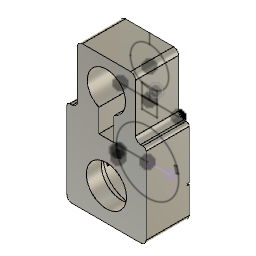
MotorEnclosure v3 (Autodesk Fusion 360 design; units mm, degrees)
Autodesk Fusion 360 part; units mm, degrees
sketch "Sketch1" plane through (0, 0, 0) normal (0, 0, 1) x (1, 0, 0)
  line L0 (-29, 0) -> (29, 0)
  line L1 (29, 0) -> (29, -17)
  line L2 (29, -17) -> (-29, -17)
  line L3 (-29, -17) -> (-29, 0)
  line L4 (-31, 2) -> (31, 2)
  line L5 (31, 2) -> (31, 0)
  line L6 (31, 0) -> (-31, 0)
  line L7 (-31, 0) -> (-31, 2)
  line L8 (-27.55, -17) -> (27.55, -17)
  line L9 (27.55, -17) -> (27.55, -26)
  line L10 (27.55, -26) -> (-27.55, -26)
  line L11 (-27.55, -26) -> (-27.55, -17)
  line L12 (-20, -26) -> (20, -26)
  line L13 (20, -26) -> (20, -41)
  line L14 (20, -41) -> (-20, -41)
  line L15 (-20, -41) -> (-20, -26)
  line L16 (-42.5, 22) -> (42.5, 22)
  line L17 (42.5, 22) -> (42.5, 2)
  line L18 (42.5, 2) -> (-42.5, 2)
  line L19 (-42.5, 2) -> (-42.5, 22)
  line L20 (-42.5, -41) -> (-20, -41)
  line L21 (42.5, 2) -> (42.5, 22)
  line L22 (-39.5, 2) -> (-39.5, -41)
  line L23 (20, -41) -> (39.5, -41)
  line L24 (39.5, -41) -> (39.5, 2)
  line L25 (0, 2) -> (0, 22)
  line L26 (0, 2) -> (0, -41)
  dimension "d1" = 17
  dimension "d2" = 58
  dimension "d3" = 2
  dimension "d4" = 62
  dimension "d5" = 55.1
  dimension "d6" = 9
  dimension "d7" = 15
  dimension "d8" = 40
  dimension "d9" = 85
  dimension "d10" = 20
  dimension "d23" = 3
  dimension "d24" = 3
  constraint horizontal L0
  constraint vertical L1
  constraint horizontal L2
  constraint vertical L3
  constraint horizontal L4
  constraint vertical L5
  constraint horizontal L6
  constraint vertical L7
  constraint midpoint origin L0
  constraint midpoint origin L6
  constraint horizontal L8
  constraint vertical L9
  constraint horizontal L10
  constraint vertical L11
  constraint coincident L2 L8.start
  constraint horizontal L12
  constraint vertical L13
  constraint horizontal L14
  constraint vertical L15
  constraint coincident L10 L12.start
  constraint horizontal L16
  constraint vertical L17
  constraint horizontal L18
  constraint vertical L19
  constraint collinear L4 L18
  constraint perpendicular L15 L20
  constraint vertical L21
  constraint coincident L18 L22.start
  constraint coincident L20 L22.end
  constraint perpendicular L20 L22
  constraint perpendicular L13 L23
  constraint coincident L18 L24.end
  constraint perpendicular L18 L24
  constraint midpoint L4 L25.start
  constraint midpoint L16 L25.end
  constraint perpendicular L4 L25
  constraint symmetric L13 L15 L25
  constraint symmetric L9 L11 L25
  constraint midpoint L14 L26.end
  measures "d1" distance of L0.start L2.end
  measures "d2" distance of L0.start L0.end
  measures "d3" distance of L4.start L6.end
  measures "d4" distance of L4.start L4.end
  measures "d5" distance of L9.end L10.end
  measures "d6" distance of L8.start L10.end
  measures "d7" distance of L12.start L14.end
  measures "d8" distance of L13.end L14.end
  measures "d9" distance of L17.end L18.end
  measures "d10" distance of L16.start L18.end
  measures "d23" distance of L19 L22
  measures "d24" distance of L21 L24
extrude "Extrude3" add sketch "Sketch1" along normal mid plane 65 contours L0 L4 L6 L7 L18 L26 | L0 L2 L3 L6 L8 L26 | L2 L3 L6 L7 L10 L11 L15 L18 L20 L22 | L0 L4 L5 L6 L18 L26 | L0 L1 L2 L6 L8 L26 | L1 L2 L5 L6 L9 L10 L13 L18 L23 L24 | L2 L8 L10 L11 L12 L26 | L2 L8 L9 L10 L12 L26 | L10 L12 L14 L15 L26 | L10 L12 L13 L14 L26
revolve "Revolve2" cut sketch "Sketch1" angle 360 about axis through (0, 2, 0) along (0, -1, 0) contours L0 L4 L6 L7 L18 L26 | L0 L2 L3 L6 L8 L26 | L2 L8 L10 L11 L12 L26 | L10 L12 L14 L15 L26
sketch "Sketch2" plane through (0, 2, 0) normal (0, 1, 0) x (-1, 0, 0)
  circle A0 centre (0, 0) radius 31
  line L0 (39.5, -32.5) -> (39.5, 32.5)
  line L1 (39.5, 32.5) -> (-39.5, 32.5)
  line L2 (-39.5, 32.5) -> (-39.5, -32.5)
  line L3 (-39.5, -32.5) -> (39.5, -32.5)
  line L4 (-39.5, 0.75) -> (-30.9909, 0.75)
  line L5 (-30.9909, 0.75) -> (-30.9909, -0.75)
  line L6 (-30.9909, -0.75) -> (-39.5, -0.75)
  line L7 (-39.5, -0.75) -> (-39.5, 0.75)
  line L8 (39.5, 0.75) -> (30.9909, 0.75)
  line L9 (30.9909, 0.75) -> (30.9909, -0.75)
  line L10 (30.9909, -0.75) -> (39.5, -0.75)
  line L11 (39.5, -0.75) -> (39.5, 0.75)
  line L12 (42.5, 0) -> (-42.5, 0)
  point P0 (28.9828, 11)
  dimension "d28" = 1.5
  dimension "d29" = 1.5
  constraint horizontal L4
  constraint vertical L5
  constraint horizontal L6
  constraint vertical L7
  constraint coincident A0 L5.end
  constraint coincident L2 L4.start
  constraint horizontal L8
  constraint vertical L9
  constraint horizontal L10
  constraint vertical L11
  constraint coincident A0 L9.end
  constraint coincident L0 L8.start
  constraint symmetric L8 L10 L12
  constraint symmetric L4 L6 L12
  constraint coincident A0 P0
  measures "d28" distance of L8 L10
  measures "d29" distance of L4 L6
extrude "Extrude4" cut sketch "Sketch2" against normal blind 2 contours A0 L0 L10 L11 L12 | A0 L0 L8 L11 L12 | A0 L2 L4 L7 L12 | A0 L2 L6 L7 L12
sketch "Sketch3" plane through (0, 0, 0) normal (0, 1, 0) x (-1, 0, 0)
  circle A0 centre (0, 0) radius 29
  arc A1 (30.9909, 0.75) -> (-30.9909, 0.75) centre (0, 0) ccw
  line L0 (-30.9909, 0.75) -> (-39.5, 0.75)
  line L1 (-39.5, 0.75) -> (-39.5, -0.75)
  line L2 (-39.5, -0.75) -> (-30.9909, -0.75)
  arc A2 (-30.9909, -0.75) -> (30.9909, -0.75) centre (0, 0) ccw
  line L3 (30.9909, -0.75) -> (39.5, -0.75)
  line L4 (39.5, -0.75) -> (39.5, 0.75)
  line L5 (39.5, 0.75) -> (30.9909, 0.75)
  line L6 (28.9828, -11) -> (30.5941, -5)
  line L7 (30.5941, -5) -> (28.6521, -4.4785)
  line L8 (28.6521, -4.4785) -> (27.0407, -10.4785)
  line L9 (27.0407, -10.4785) -> (28.9828, -11)
  line L10 (-1.75, 0) -> (-22.5, 0)
  circle A3 centre (0, 0) radius 31
  line L11 (-30.5941, 5) -> (-28.6521, 4.4785)
  line L12 (-28.9828, 11) -> (-30.5941, 5)
  line L13 (-28.6521, 4.4785) -> (-27.0407, 10.4785)
  line L14 (-27.0407, 10.4785) -> (-28.9828, 11)
  line L15 (31, 0) -> (30.5941, -5)
  line L16 (0, 0) -> (31, 0)
  dimension "d35" = 6
  dimension "d37" = 360
  dimension "d41" = 5
  constraint coincident A1 L6.start
  constraint coincident A1 L6.end
  constraint perpendicular L7 L8
  constraint perpendicular L6 L9
  constraint perpendicular L8 L9
  constraint concentric A0 A3
  constraint coincident L6.end A3
  constraint coincident A0 L7.end
  constraint coincident A3 L15.start
  constraint coincident A0.centre A1.centre
  constraint perpendicular L4 L16
  measures "d35" vertical distance of L6.start L6.end
  measures "d41" vertical distance of L6.end L15.start
extrude "Extrude5" cut sketch "Sketch3" against normal blind 13 contours A0 L11 L12 L14 | A0 L6 L7 L9
ref_plane "WorkPlane3" through (0, -9, 0) normal (0, 1, 0) x (0, 0, 1)
sketch "Sketch4" plane through (0, -9, 0) normal (0, 1, 0) x (1, 0, 0)
extrude "Extrude6" add 1 faces at (-13.1667, -26.6667, 32.5) along direction (0, 0, 1) blind 20
sketch "Sketch6" plane through (0, 0, 52.5) normal (0, 0, 1) x (-1, 0, 0)
  line L0 (39.5, 41) -> (-39.5, 41)
  line L1 (-39.5, 41) -> (-39.5, -2)
  line L2 (-39.5, -2) -> (39.5, -2)
  line L3 (39.5, -2) -> (39.5, 41)
  line L4 (-29.05, 41) -> (29.05, 41)
  line L5 (29.05, 41) -> (29.05, -2)
  line L6 (29.05, -2) -> (-29.05, -2)
  line L7 (-29.05, -2) -> (-29.05, 41)
  line L8 (29.05, 30) -> (39.5, 30)
  line L9 (-39.5, 30.6348) -> (-29.05, 30.6348)
  dimension "d44" = 58.1
  constraint horizontal L4
  constraint vertical L5
  constraint horizontal L6
  constraint vertical L7
  constraint coincident L2 L5.end
  constraint coincident L0 L4.start
  constraint coincident L5 L8.start
  constraint coincident L3 L8.end
  constraint perpendicular L3 L8
  constraint coincident L1 L9.start
  constraint coincident L7 L9.end
  constraint perpendicular L7 L9
  constraint equal L8 L9
  measures "d44" distance of L5 L7
extrude "Extrude7" add sketch "Sketch6" along normal blind 58.1 contours L0 L2 L4 L5 L6 L7
sketch "Sketch7" plane through (0, 2, 0) normal (0, 1, 0) x (-1, 0, 0)
  line L0 (-39.5, 0.75) -> (-30.9909, 0.75)
  arc A0 (30.9909, 0.75) -> (-30.9909, 0.75) centre (0, 0) ccw
  line L1 (30.9909, 0.75) -> (39.5, 0.75)
  line L2 (39.5, 0.75) -> (39.5, 52.5)
  line L3 (39.5, 52.5) -> (29.05, 52.5)
  line L4 (29.05, 52.5) -> (29.05, 110.6)
  line L5 (29.05, 110.6) -> (-29.05, 110.6)
  line L6 (-29.05, 110.6) -> (-29.05, 52.5)
  line L7 (-29.05, 52.5) -> (-39.5, 52.5)
  line L8 (-39.5, 52.5) -> (-39.5, 0.75)
  line L9 (-29.05, 52.5) -> (29.05, 52.5)
  circle A1 centre (0, 81.55) radius 19.05
  line L10 (-7.5, 64.0385) -> (7.5, 64.0385)
  line L11 (7.5, 64.0385) -> (7.5, 52.5)
  line L12 (7.5, 52.5) -> (-7.5, 52.5)
  line L13 (-7.5, 52.5) -> (-7.5, 64.0385)
  line L14 (0, 110.6) -> (0, 100.6)
  line L15 (0, 62.5) -> (0, 52.5)
  line L16 (-7.5, 52.5) -> (7.5, 52.5)
  line L17 (7.5, 52.5) -> (7.5, 40.9615)
  line L18 (7.5, 40.9615) -> (-7.5, 40.9615)
  line L19 (-7.5, 40.9615) -> (-7.5, 52.5)
  point P0 (0, 52.5)
  point P1 (-6.1183, 63.5093)
  dimension "d47" = 38.1
  dimension "d58" = 15
  constraint coincident L6.end L7.start
  constraint coincident L3.end L4.start
  constraint midpoint L9 P0
  constraint horizontal L10
  constraint vertical L11
  constraint horizontal L12
  constraint vertical L13
  constraint coincident L9 L11.end
  constraint coincident A1 L10.start
  constraint coincident A1 L10.end
  constraint midpoint L5 L14.start
  constraint coincident A1 L14.end
  constraint perpendicular L5 L14
  constraint coincident A1 P1
  constraint coincident A1 L15.start
  constraint coincident P0 L15.end
  constraint equal L14 L15
  constraint collinear L14 L15
  constraint coincident A1.centre L14
  constraint horizontal L16
  constraint vertical L17
  constraint horizontal L18
  constraint vertical L19
  constraint collinear L11 L17
  constraint equal L11 L17
  measures "d47" diameter of A1
  measures "d58" distance of L11 L13
extrude "Extrude8" cut sketch "Sketch7" against normal up to surface (43 mm away) contours A1 L10 | A1 L10
fillet "Fillet1" radius 5 1 edges at (29.05, -19.5, 52.5)
fillet "Fillet2" radius 5 1 edges at (-29.05, -19.5, 52.5)
fillet "Fillet3" radius 5 4 edges at (-29.05, -19.5, 110.6) (29.05, -19.5, 110.6) (39.5, -19.5, -32.5) (-39.5, -19.5, -32.5)
fillet "Fillet4" radius 3 2 edges at (39.5, -19.5, 52.5) (-39.5, -19.5, 52.5)
extrude "Extrude9" cut sketch "Sketch7" against normal up to surface (43 mm away) contours L9 A1 L12 L13 L15 L16 | L9 L12 L16 L17 L18 L19 | L9 A1 L11 L12 L15 L16
equation "d44 = 1.5 in + 2 cm"
equation "d45 = 1.5 in + 2 cm"
